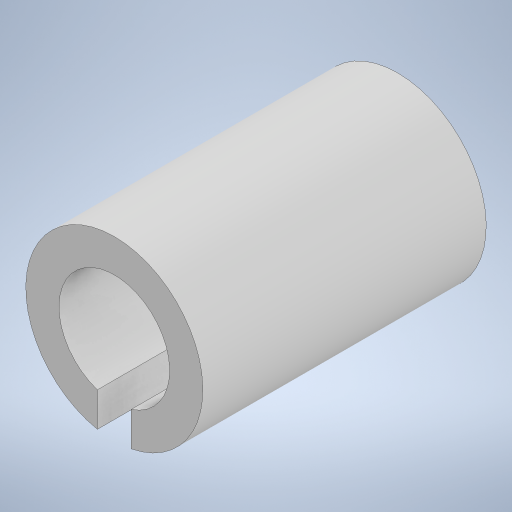
# Autodesk Inventor part: Conn Rod Crank Connector
Saved by Autodesk Inventor 2023 (Build 270158000, 158)
## iProperties
Created: 2023-02-24
Part Number: Conn Rod Crank Connector
Material: Generic
Document SubType Name: Modeling
Designer: tommy
Density: 1 g/cm^3
Appearance: Default
Author: tommy
Autodesk Inventor part; units mm, degrees
ref_plane "YZ Plane" through (0, 0, 0) normal (1, 0, 0) x (0, 1, 0)
ref_plane "XZ Plane" through (0, 0, 0) normal (0, 1, 0) x (-1, 0, 0)
ref_plane "XY Plane" through (0, 0, 0) normal (0, 0, 1) x (1, 0, 0)
sketch "Sketch1" plane through (0, 0, 0) normal (0, 0, 1) x (1, 0, 0)
  circle A0 centre (0, 0) radius 1.5875
  circle A1 centre (0, 0) radius 0.9922
  line L0 (0.3034, -0.9446) -> (0.3034, -1.5582)
  line L1 (-0.3034, -0.9446) -> (-0.3034, -1.5582)
  dimension "d0" = 3.175
  dimension "d1" = 1.9844
  constraints: 4 end point, 4 point on circle, 2 centre point, 2 coincident, 1 parallel, 1 vertical
  measures "d0" diameter of A0
  measures "d1" diameter of A1
extrude "Extrusion1" add sketch "Sketch1" along normal blind 5.08 contours A0 L0 A1 L1 picked at (1.3742, 0.1247)
body "Solid1"
